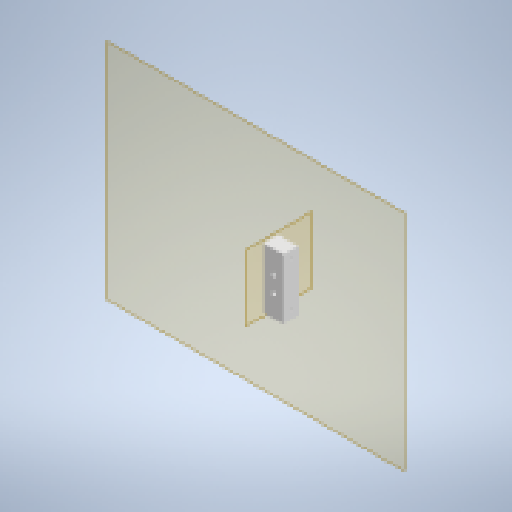
# Autodesk Inventor part: крепление
Saved by Autodesk Inventor 2024.2 (Build 282272000, 272)
## iProperties
Created: 2026-01-11
Part Number: крепление
Material: Типовые
Document SubType Name: Modeling
Designer: katya_notebook
Density: 1 g/cm^3
Appearance: По умолчанию
Author: katya_notebook
Autodesk Inventor part; units mm, degrees
ref_plane "YZ Plane" through (0, 0, 0) normal (1, 0, 0) x (0, 1, 0)
ref_plane "XZ Plane" through (0, 0, 0) normal (0, 1, 0) x (-1, 0, 0)
ref_plane "XY Plane" through (0, 0, 0) normal (0, 0, 1) x (1, 0, 0)
ref_plane "РабПлоскость1" through (0, 0, 0) normal (0, 0, 1) x (1, 0, 0)
sketch "Эскиз1" plane through (0, 0, 0) normal (0, 0, 1) x (1, 0, 0)
  circle A0 centre (32.975, 7.8539) radius 2 projected
  circle A1 centre (32.975, -8.1461) radius 2 projected
  line L0 (22.5, 91.5) -> (22.5, -91.5) projected
  line L1 (42.5, -30) -> (22.5, -30)
  line L2 (22.5, -30) -> (22.5, 30)
  line L3 (22.5, 30) -> (42.5, 30)
  line L4 (42.5, 30) -> (42.5, -30)
  line L5 (42.5, -30) -> (22.5, 30) construction
  line L6 (22.5, -30) -> (42.5, 30) construction
  point P0 (0, 0)
  point P1 (32.5, 0)
  point P2 (32.5, 0)
  point P3 (22.5, -30)
  dimension "d0" = 20
  dimension "d1" = 60
  dimension "d2" = 0
  constraints: 12 end point, 2 midpoint, 2 parallel, 1 horizontal, 1 perpendicular, 1 point on line, 1 other
  measures "d0" distance of L1.start L1.end
  measures "d1" distance of L3.end L1.start
  measures "d2" distance of point (32.5, 0) point (32.5, 0)
extrude "Выдавливание1" add sketch "Эскиз1" along normal blind 15
ref_plane "РабПлоскость2" through (22.5, -0.0677, -0.25) normal (1, 0, 0) x (0, -1, 0)
sketch "Эскиз2" plane through (22.5, -0.0677, -0.25) normal (1, 0, 0) x (0, -1, 0)
  circle A0 centre (-22.2216, -7.5) radius 1.2 projected
  circle A1 centre (22.3784, -7.5) radius 1.2 projected
  point P0 (-0.0677, -0.25)
extrude "Выдавливание2" cut sketch "Эскиз2" along normal up to surface (20 mm away)
